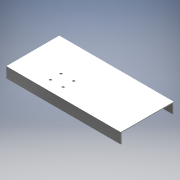
# Autodesk Inventor part: Spacer Extrusion
Saved by Autodesk Inventor 2019 (Build 230136000, 136)
## iProperties
Created: 2019-10-20
Part Number: Spacer Extrusion
Material: Aluminum 6061
Document SubType Name: Modeling
Designer: admin
Density: 2.7 g/cm^3
Appearance: Aluminum - Flat
Author: admin
Autodesk Inventor part; units mm, degrees
ref_plane "YZ Plane" through (0, 0, 0) normal (1, 0, 0) x (0, 1, 0)
ref_plane "XZ Plane" through (0, 0, 0) normal (0, 1, 0) x (-1, 0, 0)
ref_plane "XY Plane" through (0, 0, 0) normal (0, 0, 1) x (1, 0, 0)
sketch "Sketch1" plane through (0, 0, 0) normal (1, 0, 0) x (0, 1, 0)
  line L0 (0, 0) -> (25, 0)
  line L1 (25, 0) -> (25, -125)
  line L2 (25, -125) -> (0, -125)
  line L3 (0, -125) -> (0, -123)
  line L4 (0, -123) -> (23, -123)
  line L5 (23, -123) -> (23, -2)
  line L6 (23, -2) -> (0, -2)
  line L7 (0, -2) -> (0, 0)
  dimension "d0" = 2
  dimension "d1" = 2
  dimension "d2" = 125
  dimension "d3" = 25
  dimension "d4" = 2
  constraints: 16 end point, 7 perpendicular, 1 horizontal, 1 point on line
  measures "d0" distance of L6.end L0.start
  measures "d1" distance of L2.end L3.end
  measures "d2" distance of L0.end L1.end
  measures "d3" distance of L0.start L0.end
  measures "d4" distance between parallel lines of L1 L5
extrude "Extrusion1" add sketch "Sketch1" along normal blind 200 and the other way blind 70
sketch "Sketch2" plane through (-70, 25, 0) normal (0, 1, 0) x (1, 0, 0)
  circle A0 centre (80, 24) radius 2.75
  circle A1 centre (80, 49) radius 2.75
  circle A2 centre (110, 24) radius 2.75
  circle A3 centre (110, 49) radius 2.75
  line L0 (0, 0) -> (0, 125) projected
  line L1 (270, 0) -> (0, 0) projected
  circle A4 centre (9.057, 107.86) radius 2.65
  circle A5 centre (9.057, 93.86) radius 2.65
  circle A6 centre (39.057, 107.86) radius 2.65
  circle A7 centre (39.057, 93.86) radius 2.65
  line L2 (270, 125) -> (0, 125) projected
  point P0 (70, 0)
  dimension "d9" = 5.5
  dimension "d10" = 5.5
  dimension "d11" = 5.5
  dimension "d12" = 5.5
  dimension "d13" = 80
  dimension "d14" = 80
  dimension "d15" = 24
  dimension "d16" = 110
  dimension "d17" = 110
  dimension "d18" = 24
  dimension "d19" = 25
  dimension "d20" = 25
  dimension "d23" = 5.3
  dimension "d24" = 5.3
  dimension "d25" = 5.3
  dimension "d26" = 5.3
  dimension "d27" = 9.057
  dimension "d28" = 9.057
  dimension "d29" = 14
  dimension "d30" = 30
  dimension "d31" = 30
  dimension "d32" = 14
  dimension "d33" = 30
  dimension "d34" = 14
  dimension "d36" = 17.14
  constraints: 8 centre point
  measures "d9" diameter of A0
  measures "d10" diameter of A1
  measures "d11" diameter of A2
  measures "d12" diameter of A3
  measures "d13" distance from line of L0 A1.centre
  measures "d14" distance from line of L0 A0.centre
  measures "d15" distance from line of L1 A2.centre
  measures "d16" distance from line of A3.centre L0
  measures "d17" distance from line of L0 A2.centre
  measures "d18" distance from line of L1 A0.centre
  measures "d19" distance of A0.centre A1.centre
  measures "d20" distance of A2.centre A3.centre
  measures "d23" diameter of A4
  measures "d24" diameter of A5
  measures "d25" diameter of A6
  measures "d26" diameter of A7
  measures "d27" distance from line of L0 A5.centre
  measures "d28" distance from line of L0 A4.centre
  measures "d29" distance of A5.centre A4.centre
  measures "d30" distance of A6.centre A4.centre
  measures "d31" distance of A5.centre A7.centre
  measures "d32" vertical distance of A4.centre A7.centre
  measures "d33" horizontal distance of A5.centre A6.centre
  measures "d34" distance of A7.centre A6.centre
  measures "d36" distance from line of L2 A4.centre
extrude "Extrusion2" cut sketch "Sketch2" against normal blind 10
body "Solid1"
